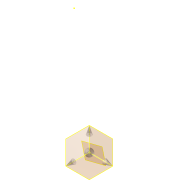
# Autodesk Inventor part: Agarre Cortadora
Saved by Autodesk Inventor 2021 (Build 250183000, 183)
## iProperties
Created: 2021-07-14
Part Number: Agarre Cortadora
Material: Stainless Steel, Polished
Document SubType Name: Modeling
Designer: maaro
Density: 8 g/cm^3
Appearance: Stainless - Polished
Mass: 3277.4 g
Surface Area: 877.022 cm^2
Volume: 409.676 cm^3
Author: maaro
Autodesk Inventor part; units mm, degrees
ref_plane "YZ Plane" through (0, 0, 0) normal (1, 0, 0) x (0, 1, 0)
ref_plane "XZ Plane" through (0, 0, 0) normal (0, 1, 0) x (-1, 0, 0)
ref_plane "XY Plane" through (0, 0, 0) normal (0, 0, 1) x (1, 0, 0)
ref_plane "Work Plane1" through (838.3238, -6744.4303, 0) normal (0, 0, 1) x (-0.9694, -0.2455, 0)
sketch "Sketch1" plane through (838.3238, -6744.4303, 0) normal (0, 0, 1) x (-0.9694, -0.2455, 0)
  circle A0 centre (0, 0) radius 35
  circle A1 centre (0, 0) radius 25
  arc A2 (-5.7334, 13.861) -> (-0.8591, 14.9754) centre (0, 0) ccw
  line L0 (-0.8591, 14.9754) -> (-2.9117, 23.9535)
  line L1 (-2.9117, 23.9535) -> (1.4752, 24.9564)
  arc A3 (-12.1727, 21.8363) -> (1.4752, 24.9564) centre (0, 0) ccw
  line L2 (-12.1727, 21.8363) -> (-7.7859, 22.8392)
  line L3 (-7.7859, 22.8392) -> (-5.7334, 13.861)
  point P0 (-843.1619, -6743.8271)
  dimension "d0" = 70
  dimension "d1" = 50
  constraints: 8 end point, 4 centre point, 4 point on circle, 1 coincident, 1 concentric, 14 other
  measures "d0" diameter of A0
  measures "d1" diameter of A1
extrude "Extrusion1" add sketch "Sketch1" along normal mid plane 150
sketch "Sketch2" plane through (838.3238, -6744.4303, 0) normal (0, 0, 1) x (-0.9694, -0.2455, 0)
  point P0 (-843.1619, -6743.8271)
sketch "Sketch3" plane through (838.3238, -6744.4303, 0) normal (0, 0, 1) x (-0.9694, -0.2455, 0)
  circle A0 centre (0, 0) radius 35 projected
  arc A1 (-11.9707, 32.8892) -> (-31.7208, 14.7916) centre (0, 0) ccw
  line L0 (0, 0) -> (-11.9707, 32.8892) construction
  line L1 (0, 0) -> (35, 0) construction
  line L2 (0, 0) -> (-31.7208, 14.7916) construction
  line L3 (-11.9707, 32.8892) -> (-31.7208, 14.7916) construction
  line L4 (-11.9707, 32.8892) -> (-147.0887, 180.3447)
  line L5 (-147.0887, 180.3447) -> (-166.8388, 162.2471)
  line L6 (-166.8388, 162.2471) -> (-31.7208, 14.7916)
  circle A2 centre (-129.1006, 140.8886) radius 5 projected
  point P0 (-843.1619, -6743.8271)
  point P1 (-156.9638, 171.2959)
  dimension "d4" = 35
  dimension "d5" = 110
  dimension "d6" = 45
  dimension "d8" = 200
  constraints: 14 end point, 4 point on circle, 2 perpendicular, 1 centre point, 1 equal length, 1 horizontal, 1 midpoint, 1 parallel
  measures "d4" radius of A1
  measures "d5" angle of L1 L0
  measures "d6" angle of L0 L2
  measures "d8" distance of L5.end L2.end
extrude "Extrusion2" add sketch "Sketch3" along normal mid plane 30 contours A0 L6 L5 L4
body "Solid1"
